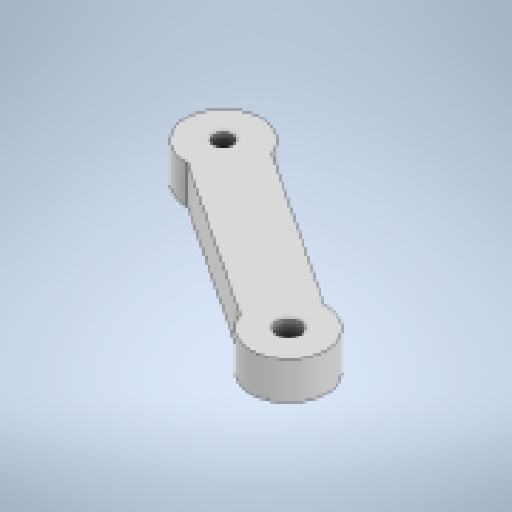
# Autodesk Inventor part: gripper_hand_connector
Saved by Autodesk Inventor 2024 (Build 280153000, 153)
## iProperties
Created: 2023-09-08
Part Number: gripper_hand_connector
Material: Generic
Document SubType Name: Modeling
Designer: 박동준
Density: 1 g/cm^3
Appearance: Default
Author: 박동준
Autodesk Inventor part; units mm, degrees
ref_plane "YZ Plane" through (0, 0, 0) normal (1, 0, 0) x (0, 1, 0)
ref_plane "XZ Plane" through (0, 0, 0) normal (0, 1, 0) x (-1, 0, 0)
sketch "Sketch1" plane through (0, 0, 0) normal (0, 1, 0) x (-1, 0, 0)
  circle A0 centre (0, 0) radius 5
  circle A1 centre (-25.7936, 17.1957) radius 5
  line L0 (-4.715, -1.6641) -> (-25.5162, 12.2034)
  line L1 (-0.2774, 4.9923) -> (-21.0786, 18.8598)
  line L2 (0, 0) -> (-25.7936, 0) construction
  line L3 (-25.7936, 0) -> (-25.7936, 17.1957) construction
  line L4 (0, 0) -> (-25.7936, 17.1957) construction
  dimension "d0" = 10
  dimension "d1" = 10
  dimension "d2" = 4
  dimension "d3" = 4
  dimension "d27" = 25
  dimension "d28" = 33.69
  constraints: 10 end point, 4 point on circle, 2 centre point, 2 parallel, 1 coincident, 1 horizontal, 1 perpendicular
  measures "d0" diameter of A0
  measures "d1" diameter of A1
  measures "d2" distance between parallel lines of L0 L4
  measures "d3" distance between parallel lines of L1 L4
  measures "d27" distance of L0.start L0.end
  measures "d28" angle of L2 L0
extrude "Extrusion1" add sketch "Sketch1" along normal blind 5
sketch "Sketch2" plane through (0, 0, 0) normal (0, -1, 0) x (1, 0, 0)
  line L0 (0, 0) -> (25.7936, 17.1957) construction
  arc A0 (25.5162, 12.2034) -> (21.0786, 18.8598) centre (25.7936, 17.1957) ccw projected
  line L1 (0.2774, 4.9923) -> (21.0786, 18.8598) projected
  arc A1 (0.2774, 4.9923) -> (4.715, -1.6641) centre (0, 0) ccw projected
  line L2 (25.5162, 12.2034) -> (4.715, -1.6641) projected
  constraints: 2 coincident
hole "Hole1" at (25.7936, 0, 17.1957) direction (0, 1, 0) diameter 3.1 end through all
ref_plane "Work Plane1" through (0, 1.5, 0) normal (0, 1, 0) x (1, 0, 0)
sketch "Sketch4" plane through (0, 5, 0) normal (0, 1, 0) x (1, 0, 0)
  circle A0 centre (25.7936, -17.1957) radius 1.55 projected
  arc A1 (21.0786, -18.8598) -> (25.5162, -12.2034) centre (25.7936, -17.1957) ccw projected
  line L0 (25.5162, -12.2034) -> (4.715, 1.6641) projected
  arc A2 (4.715, 1.6641) -> (0.2774, -4.9923) centre (0, 0) ccw projected
  line L1 (0.2774, -4.9923) -> (21.0786, -18.8598) projected
  constraints: 1 coincident
hole "Hole2" at (0, 5, 0) direction (0, -1, 0) diameter 2.459 end through all thread size "M3x0.5" class "6H" standard "ISO Metric profile"
body "Solid1"
